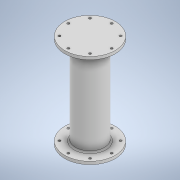
# Autodesk Inventor part: Connection_link_1
Saved by Autodesk Inventor 2021 (Build 250183000, 183)
## iProperties
Created: 2020-05-19
Part Number: Connection_link_1
Material: Generic
Document SubType Name: Modeling
Designer: Motius
Density: 1 g/cm^3
Appearance: Default
Author: Motius
Autodesk Inventor part; units mm, degrees
ref_plane "YZ Plane" through (0, 0, 0) normal (1, 0, 0) x (0, 1, 0)
ref_plane "XZ Plane" through (0, 0, 0) normal (0, 1, 0) x (-1, 0, 0)
ref_plane "XY Plane" through (0, 0, 0) normal (0, 0, 1) x (1, 0, 0)
sketch "Sketch1" plane through (0, 0, 0) normal (0, 0, 1) x (1, 0, 0)
  line L0 (0, 91) -> (0, -91) construction
  line L1 (-7, 0) -> (42, 0) construction
  line L2 (0, -65) -> (0, 65)
  line L3 (0, -65) -> (35, -65)
  line L4 (35, -65) -> (35, 65)
  line L5 (35, 65) -> (0, 65)
  point P0 (0, 0)
  dimension "d2" = 130
  dimension "d12" = 35
  constraints: 8 end point, 1 collinear, 1 perpendicular, 1 vertical, 1 other
  measures "d2" distance of L3.end L4.end
  measures "d12" distance between parallel lines of L4 L0
revolve "Revolution1" add sketch "Sketch1" angle 360 about axis through (0, 0, 0) along (0, -1, 0)
sketch "Sketch4" plane through (0, 0, 0) normal (0, 0, 1) x (1, 0, 0)
  line L0 (-35, 65) -> (35, 65) construction
  line L1 (-35, -65) -> (35, -65) construction
  line L2 (0, 91) -> (0, -91) construction
  line L3 (-49, 0) -> (49, 0) construction
  line L4 (35, -61) -> (22, -61)
  line L5 (20, -59) -> (20, 59)
  line L6 (22, 61) -> (35, 61)
  line L7 (35, 65) -> (35, -65) construction
  line L8 (35, -61) -> (35, 61)
  arc A0 (20, -59) -> (22, -61) centre (22, -59) ccw
  arc A1 (22, 61) -> (20, 59) centre (22, 59) ccw
  point P0 (0, 0)
  dimension "d35" = 20
  dimension "d36" = 4
  dimension "d37" = 2
  constraints: 8 end point, 4 point on circle, 4 tangent, 2 centre point, 2 perpendicular, 1 collinear, 1 equal radius, 1 horizontal, 1 point on line, 1 other
  measures "d35" distance between parallel lines of L2 L5
  measures "d36" distance between parallel lines of L1 L4
  measures "d37" radius of A0
revolve "Revolution2" cut sketch "Sketch4" angle 360 about axis through (0, 0, 0) along (0, -1, 0)
sketch "Sketch2" plane through (0, 65, 0) normal (0, -1, 0) x (1, 0, 0)
  circle A0 centre (0, 0) radius 35 construction
  line L0 (-49, 0) -> (49, 0) construction
  line L1 (0, 49) -> (0, -49) construction
  circle A1 centre (0, 0) radius 21.25 construction
  circle A2 centre (0, 0) radius 30 construction
  point P0 (0, 30)
  point P1 (0, 21.25)
  point P2 (-21.2132, 21.2132)
  point P3 (-15.026, 15.026)
  point P4 (-30, 0)
  point P5 (-21.25, 0)
  point P6 (-21.2132, -21.2132)
  point P7 (-15.026, -15.026)
  point P8 (0, -30)
  point P9 (0, -21.25)
  point P10 (21.2132, -21.2132)
  point P11 (15.026, -15.026)
  point P12 (30, 0)
  point P13 (21.25, 0)
  point P14 (21.2132, 21.2132)
  point P15 (15.026, 15.026)
  dimension "d6" = 42.5
  dimension "d7" = 60
  dimension "d10" = 360
  constraints: 2 coincident, 2 point on line, 2 vertical alignment, 21 other
hole "Hole2" at (0, 65, 30) at (-21.2132, 65, 21.2132) at (-30, 65, 0) at (-21.2132, 65, -21.2132) at (0, 65, -30) at (21.2132, 65, -21.2132) at (30, 65, 0) at (21.2132, 65, 21.2132) direction (0, -1, 0) diameter 3.242 depth 4 tip angle 118 thread size "M4x0.7" class "6H" standard "ANSI Metric M Profile"
mirror "Mirror1" about plane through (0, 0, 0) normal (0, 1, 0) of "Hole2"
body "Solid1"
